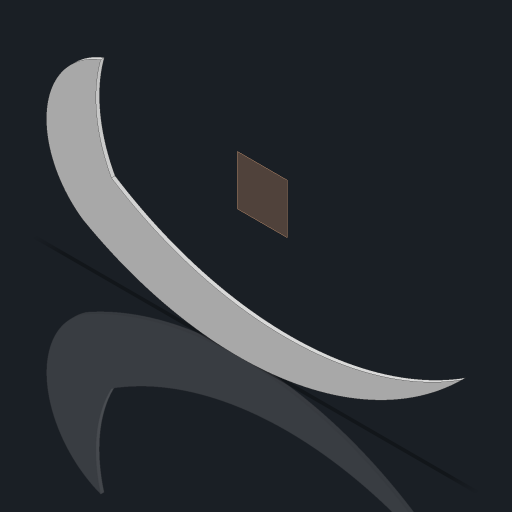
# Autodesk Inventor part: Triball Holder
Saved by Autodesk Inventor 2023.2 (Build 272271030, 271C)
## iProperties
Created: 2024-03-28
Part Number: Triball Holder
Material: Generic
Document SubType Name: Modeling
Designer: Michael
Density: 1 g/cm^3
Appearance: Default
Author: Michael
Autodesk Inventor part; units mm, degrees
ref_plane "YZ Plane" through (0, 0, 0) normal (1, 0, 0) x (0, 1, 0)
ref_plane "XZ Plane" through (0, 0, 0) normal (0, 1, 0) x (-1, 0, 0)
ref_plane "XY Plane" through (0, 0, 0) normal (0, 0, 1) x (1, 0, 0)
ref_plane "Work Plane1" through (0, 0, 1.5875) normal (0, 0, 1) x (1, 0, 0)
sketch "Sketch2" plane through (0, 0, 1.5875) normal (0, 0, 1) x (1, 0, 0)
  arc A0 (-69.85, 17.4625) -> (-65.0875, -25.4) centre (-14.3813, 1.9299) ccw
  arc A1 (-65.0875, -25.4) -> (89.8524, -25.2442) centre (12.2604, 96.064) ccw
  arc A2 (-69.85, 17.4625) -> (-77.7875, -47.625) centre (-56.8771, -17.1473) ccw
  arc A3 (-77.7875, -47.625) -> (89.8524, -25.2442) centre (-8.8035, 74.6915) ccw
  point P0 (0, 0)
  dimension "d4" = 154.94
  constraints: 8 point on circle, 4 centre point
  measures "d4" distance of A0.end A1.end
extrude "Extrusion2" add sketch "Sketch2" along normal blind 1.5875
body "Solid2"
